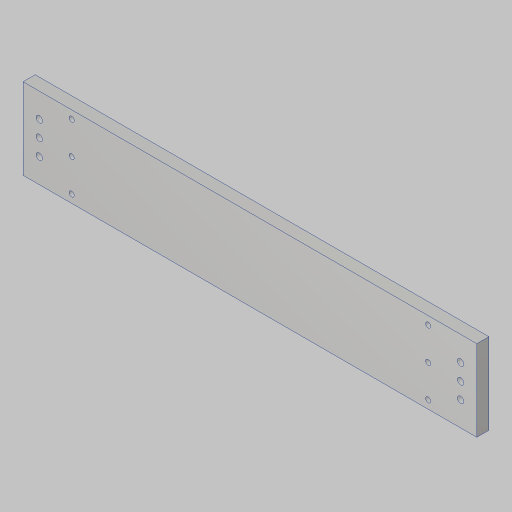
# Autodesk Inventor part: EL2-003
Saved by Autodesk Inventor 2023.5 (Build 275446000, 446)
## iProperties
Created: 2025-01-10
Part Number: EL2-003
Material: Aluminum 6061
Document SubType Name: Modeling
Designer: mavericks
Density: 2.7 g/cm^3
Appearance: Aluminum - Flat
Author: mavericks
Autodesk Inventor part; units mm, degrees
ref_plane "YZ Plane" through (0, 0, 0) normal (1, 0, 0) x (0, 1, 0)
ref_plane "XZ Plane" through (0, 0, 0) normal (0, 1, 0) x (-1, 0, 0)
ref_plane "XY Plane" through (0, 0, 0) normal (0, 0, 1) x (1, 0, 0)
sketch "Sketch1" plane through (0, 0, 0) normal (0, 0, 1) x (1, 0, 0)
  line L0 (-177.8, -31.75) -> (177.8, -31.75)
  line L1 (177.8, -31.75) -> (177.8, 31.75)
  line L2 (177.8, 31.75) -> (-177.8, 31.75)
  line L3 (-177.8, 31.75) -> (-177.8, -31.75)
  line L4 (-177.8, -31.75) -> (177.8, 31.75) construction
  line L5 (177.8, -31.75) -> (-177.8, 31.75) construction
  point P0 (0, 0)
  dimension "d0" = 355.6
  dimension "d1" = 63.5
  constraints: 12 end point, 2 midpoint, 2 parallel, 1 horizontal, 1 perpendicular
  measures "d0" distance of L2.end L1.end
  measures "d1" distance of L1.end L0.end
extrude "Extrusion1" add sketch "Sketch1" along normal blind 9.525
sketch "Sketch3" plane through (0, 0, 9.525) normal (0, 0, 1) x (1, 0, 0)
  line L0 (-177.8, 31.75) -> (-177.8, -31.75) projected
  line L1 (0, 0) -> (0, 31.75) construction
  line L2 (177.8, 31.75) -> (-177.8, 31.75) projected
  point P0 (-165.1, 12.7)
  point P1 (-165.1, -12.7)
  point P2 (-165.1, 0)
  point P3 (-177.8, 0)
  point P4 (165.1, 12.7)
  point P5 (165.1, -12.7)
  point P6 (165.1, 0)
  dimension "d9" = 12.7
  dimension "d10" = 12.7
  dimension "d11" = 12.7
  constraints: 3 symmetric about line, 2 end point, 2 midpoint, 2 vertical alignment, 1 horizontal alignment
  measures "d9" distance from line of L0 point (-165.1, 12.7)
  measures "d10" distance of point (-165.1, 0) point (-165.1, 12.7)
  measures "d11" distance of point (-165.1, -12.7) point (-165.1, 0)
hole "Hole1" at (-165.1, 12.7, 9.525) at (-165.1, -12.7, 9.525) at (-165.1, 0, 9.525) at (165.1, 0, 9.525) at (165.1, -12.7, 9.525) at (165.1, 12.7, 9.525) direction (0, 0, -1) diameter 4.9784 end through all thread size "1/4-20 UNC" class "2B" standard "ANSI Unified Screw Threads"
sketch "Sketch4" plane through (0, 0, 9.525) normal (0, 0, 1) x (1, 0, 0)
  line L0 (-139.7, 0) -> (139.7, 0) construction
  point P0 (0, 0)
  point P1 (-139.7, 25.4)
  point P2 (-139.7, -25.4)
  point P3 (139.7, 25.4)
  point P4 (139.7, -25.4)
  point P5 (0, 0)
  dimension "d19" = 25.4
  dimension "d20" = 25.4
  dimension "d21" = 279.4
  constraints: 4 horizontal alignment, 4 vertical alignment, 2 end point, 1 coincident, 1 horizontal, 1 midpoint
  measures "d19" distance of L0.start point (-139.7, 25.4)
  measures "d20" distance of point (-139.7, -25.4) L0.start
  measures "d21" distance of L0.start L0.end
hole "Hole2" at (-139.7, 25.4, 9.525) at (-139.7, 0, 9.525) at (-139.7, -25.4, 9.525) at (139.7, 25.4, 9.525) at (139.7, 0, 9.525) at (139.7, -25.4, 9.525) direction (0, 0, -1) diameter 3.9624 end through all thread size "10-32 UNF" class "2B" standard "ANSI Unified Screw Threads"
body "Solid1"
